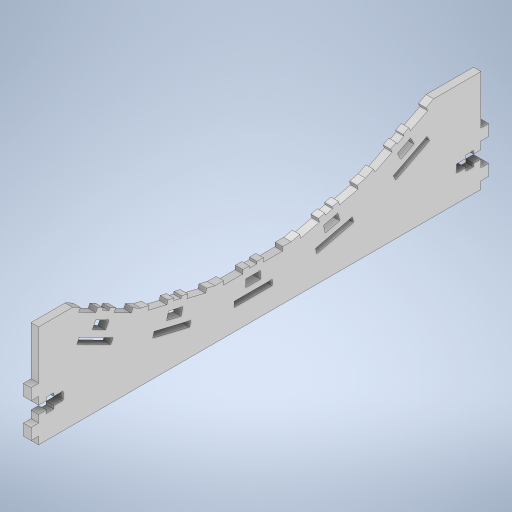
# Autodesk Inventor part: switchplate-support-03
Saved by Autodesk Inventor 2024.1 (Build 281209000, 209)
## iProperties
Created: 2019-06-27
Material: Acier, galvanisé
Document SubType Name: Modeling
Designer: Thibault
Density: 7.85 g/cm^3
Appearance: Aluminium - Poli
Mass: 11.7255 g
Surface Area: 33.7109 cm^2
Volume: 1.4937 cm^3
Part Number: switchplate-support-03
sa_0: 0.400 nd
height_shift: 0,000 mm
base_height: 27,000 mm
switchplate_depth: 121,000 mm
short_switchplate_depth: 96,505 mm
Author: Thibault
Autodesk Inventor part; units mm, degrees
ref_plane "YZ Plane" through (0, 0, 0) normal (1, 0, 0) x (0, 1, 0)
ref_plane "XZ Plane" through (0, 0, 0) normal (0, 1, 0) x (-1, 0, 0)
ref_plane "XY Plane" through (0, 0, 0) normal (0, 0, 1) x (1, 0, 0)
sketch "Anchor (nut side)" plane through (0, 0, 0) normal (0, 0, 1) x (1, 0, 0)
  line L0 (11.1, 0) -> (9.1, 0)
  line L1 (9.1, 0) -> (9.1, -2)
  line L2 (9.1, -2) -> (9.9, -2)
  line L3 (9.9, -2) -> (9.9, -4)
  line L4 (6.2, -4) -> (6.2, -2)
  line L5 (6.2, -2) -> (7, -2)
  line L6 (7, -2) -> (7, 0)
  line L7 (7, 0) -> (5, 0)
  line L8 (2, 0) -> (2, 2)
  line L9 (2, 0) -> (3, 0) construction
  line L10 (2, 2) -> (5, 2)
  line L11 (5, 2) -> (5, 0)
  line L12 (11.1, 0) -> (11.1, 2)
  line L13 (11.1, 2) -> (14.1, 2)
  line L14 (14.1, 2) -> (14.1, 0)
  line L15 (0, 0) -> (2, 0)
  line L16 (14.1, 0) -> (16.1, 0)
  line L17 (6.2, -4) -> (7, -4)
  line L18 (9.9, -4) -> (9.1, -4)
  line L19 (7, -4) -> (7, -6.25)
  line L20 (9.1, -4) -> (9.1, -6.25)
  line L21 (7.25, -6.5) -> (8.05, -6.5)
  arc A0 (7, -6.25) -> (7.25, -6.5) centre (7.25, -6.25) ccw
  arc A1 (8.85, -6.5) -> (9.1, -6.25) centre (8.85, -6.25) ccw
  line L22 (8.05, -6.5) -> (8.85, -6.5)
  line L23 (8.05, -3.8983) -> (8.05, -9.959) construction
  point P0 (9.1321, -0.6227)
  point P1 (7, -6.5)
  point P2 (9.1, -6.5)
  dimension "d3" = 2
  dimension "d7" = 6.1
  dimension "d10" = 2
  dimension "d11" = 2
  dimension "d12" = 0.8
  dimension "d13" = 2
  dimension "d14" = 0.8
  dimension "d15" = 2.1
  dimension "d18" = 2
  dimension "d19" = 0.8
  dimension "d20" = 0.8
  dimension "d21" = 2.5
  dimension "d22" = 2.5
  dimension "d23" = 2.1
  dimension "d38" = 2
  dimension "d39" = 0.25
  dimension "d120" = 3
  measures "d3" distance of point (0, 0) L8.start
  measures "d7" distance of L7.end L0.start
  measures "d10" distance of L0.start L0.end
  measures "d11" distance of L0.end L1.end
  measures "d12" distance of L1.end L2.end
  measures "d13" distance of L2.end L3.end
  measures "d14" distance of L4.end L5.end
  measures "d15" distance of L6.end L0.end
  measures "d18" distance of L14.end point (16.1, 0)
  measures "d19" distance of L4.start L17.end
  measures "d20" distance of L3.end L18.end
  measures "d21" distance of L17.end point (7, -6.5)
  measures "d22" distance of L18.end point (9.1, -6.5)
  measures "d23" distance of L17.end L18.end
  measures "d38" distance of the line from the sketch origin of L10
  measures "d39" radius of A0
  measures "d120" distance of L8.end L10.end
sketch "Anchor (screw side)" plane through (0, 0, 0) normal (0, 0, 1) x (1, 0, 0)
  circle A0 centre (93.8994, 50.2542) radius 1.05
  line L0 (90.8494, 51.2542) -> (87.8494, 51.2542)
  line L1 (87.8494, 51.2542) -> (87.8494, 49.2542)
  line L2 (87.8494, 49.2542) -> (90.8494, 49.2542)
  line L3 (90.8494, 49.2542) -> (90.8494, 51.2542)
  line L4 (99.9494, 51.2542) -> (96.9494, 51.2542)
  line L5 (96.9494, 51.2542) -> (96.9494, 49.2542)
  line L6 (96.9494, 49.2542) -> (99.9494, 49.2542)
  line L7 (99.9494, 49.2542) -> (99.9494, 51.2542)
  line L8 (90.8494, 51.2542) -> (96.9494, 49.2542) construction
  line L9 (96.9494, 51.2542) -> (90.8494, 49.2542) construction
  line L10 (85.8494, 53.2542) -> (101.9494, 53.2542) construction
  line L11 (101.9494, 53.2542) -> (101.9494, 47.2542) construction
  line L12 (101.9494, 47.2542) -> (85.8494, 47.2542) construction
  line L13 (85.8494, 47.2542) -> (85.8494, 53.2542) construction
  point P0 (103.5798, 50.1132)
  dimension "d27_1" = 2.1
  dimension "d28_1" = 3
  dimension "d29" = 2
  dimension "slot_distance" = 6.1
  dimension "d34" = 2
  dimension "d35" = 2
  dimension "d36" = 2
  dimension "d37" = 2
  measures "d27_1" diameter of A0
  measures "d28_1" distance of L2.end L1.end
  measures "d29" distance of L1.end L0.end
  measures "slot_distance" distance between parallel lines of L5 L3
  measures "d34" distance between parallel lines of L0 L10
  measures "d35" distance between parallel lines of L12 L2
  measures "d36" distance between parallel lines of L11 L7
  measures "d37" distance between parallel lines of L13 L1
sketch "Switch support" plane through (0, 0, 0) normal (0, 0, 1) x (1, 0, 0)
  line L0 (15.2854, 16.4472) -> (15.9854, 16.4472)
  line L1 (15.9854, 16.4472) -> (15.9854, 15.4472)
  line L2 (31.5854, 15.4472) -> (31.5854, 16.4472)
  line L3 (31.5854, 16.4472) -> (32.2854, 16.4472)
  line L4 (15.9854, 15.4472) -> (21.0554, 15.4472)
  line L5 (21.0554, 15.4472) -> (21.0554, 16.4472)
  line L6 (21.0554, 16.4472) -> (22.7854, 16.4472)
  line L7 (22.7854, 16.4472) -> (22.7854, 15.8972)
  line L8 (22.7854, 15.8972) -> (24.7854, 15.8972)
  line L9 (24.7854, 15.8972) -> (24.7854, 16.4472)
  line L10 (24.7854, 16.4472) -> (26.5154, 16.4472)
  line L11 (26.5154, 15.4472) -> (26.5154, 16.4472)
  line L12 (26.5154, 15.4472) -> (31.5854, 15.4472)
  line L13 (21.8354, 13.9472) -> (25.7354, 13.9472)
  line L14 (25.7354, 13.9472) -> (25.7354, 11.9472)
  line L15 (25.7354, 11.9472) -> (21.8354, 11.9472)
  line L16 (21.8354, 11.9472) -> (21.8354, 13.9472)
  line L17 (23.7854, 15.8972) -> (23.7854, 13.9472) construction
  line L18 (18.7854, 10.3472) -> (28.7854, 10.3472)
  line L19 (28.7854, 10.3472) -> (28.7854, 8.9472)
  line L20 (28.7854, 8.9472) -> (18.7854, 8.9472)
  line L21 (18.7854, 8.9472) -> (18.7854, 10.3472)
  line L22 (23.7854, 11.9472) -> (23.7854, 10.3472) construction
  point P0 (20.0288, 26.7181)
  point P1 (18.5204, 15.4472)
  dimension "d43" = 1
  dimension "d48" = 17
  dimension "d124" = 0.7
  dimension "d125" = 0.7
  dimension "d126" = 1
  dimension "d127" = 5.07
  dimension "d128" = 1
  dimension "d129" = 1.73
  dimension "d131" = 0.55
  dimension "d132" = 2
  dimension "d133" = 0.55
  dimension "d135" = 1.73
  dimension "d136" = 5.07
  dimension "d137" = 1
  dimension "d138" = 3.9
  dimension "d139" = 2
  dimension "d140" = 1.5
  dimension "d141" = 1.4
  dimension "d142" = 10
  dimension "d143" = 5.1
  measures "d43" distance of L1.start L1.end
  measures "d48" distance of point (32.285, 16.447) point (15.285, 16.447)
  measures "d124" distance of L2.end point (32.285, 16.447)
  measures "d125" distance of point (15.285, 16.447) L1.start
  measures "d126" distance of L2.start L2.end
  measures "d127" distance of L1.end L4.end
  measures "d128" distance of L4.end L5.end
  measures "d129" distance of L5.end L6.end
  measures "d131" distance of L6.end L7.end
  measures "d132" distance of L7.end L8.end
  measures "d133" distance of L8.end L9.end
  measures "d135" distance of L9.end L10.end
  measures "d136" distance of L11.start L2.start
  measures "d137" distance of L11.start L10.end
  measures "d138" distance of L14.end L15.end
  measures "d139" distance of L13.end L14.end
  measures "d140" distance between parallel lines of L13 L4
  measures "d141" distance of L20.end L18.start
  measures "d142" distance of L18.start L18.end
  measures "d143" distance from line of L18 point (18.52, 15.447)
sketch "Sketch1" plane through (0, 0, 0) normal (1, 0, 0) x (0, 1, 0)
  line L0 (0, -121) -> (27, -121)
  line L1 (27, 0) -> (0, 0)
  line L2 (27, -121) -> (27, -106.4804)
  line L3 (26.47, -12.0403) -> (27, -11)
  line L4 (28.2121, -16.9724) -> (22.1003, -16.9724)
  line L5 (26.2736, -12.4256) -> (27, -11)
  line L6 (18.5558, -27.5727) -> (17.8294, -28.9983)
  line L7 (21.9473, -35.6102) -> (15.8356, -35.6102)
  line L8 (17.4559, -30.5541) -> (17.8294, -28.9983)
  line L9 (13.4873, -47.0844) -> (13.1138, -48.6402)
  line L10 (19.8511, -55.1756) -> (13.7394, -55.1756)
  line L11 (13.1138, -50.2402) -> (13.1138, -48.6402)
  line L12 (13.1138, -67.2402) -> (13.1138, -68.8402)
  line L13 (22.0358, -74.7409) -> (15.9241, -74.7409)
  line L14 (13.4873, -70.396) -> (13.1138, -68.8402)
  line L15 (17.4559, -86.9263) -> (17.8294, -88.4821)
  line L16 (28.3566, -93.3787) -> (22.2449, -93.3787)
  line L17 (18.5558, -89.9077) -> (17.8294, -88.4821)
  line L18 (26.2736, -105.0548) -> (27, -106.4804)
  line L19 (27, 0) -> (27, -11)
  line L20 (0, 0) -> (0, -121)
  line L21 (17.4559, -30.5541) -> (17.2925, -31.2348)
  line L22 (17.2925, -31.2348) -> (16.3201, -31.0013)
  line L23 (12.6783, -46.1703) -> (13.6507, -46.4038)
  line L24 (13.6507, -46.4038) -> (13.4873, -47.0844)
  line L25 (16.3201, -31.0013) -> (15.1365, -35.9313)
  line L26 (15.1365, -35.9313) -> (16.1089, -36.1647)
  line L27 (16.1089, -36.1647) -> (15.705, -37.8469)
  line L28 (15.705, -37.8469) -> (15.1702, -37.7185)
  line L29 (15.1702, -37.7185) -> (14.7033, -39.6632)
  line L30 (14.7033, -39.6632) -> (15.2381, -39.7916)
  line L31 (15.2381, -39.7916) -> (14.8343, -41.4738)
  line L32 (13.8619, -41.2404) -> (14.8343, -41.4738)
  line L33 (13.8619, -41.2404) -> (12.6783, -46.1703)
  line L34 (13.4959, -36.3395) -> (12.5855, -40.1318)
  line L35 (12.5855, -40.1318) -> (10.6407, -39.6649)
  line L36 (10.6407, -39.6649) -> (11.5511, -35.8726)
  line L37 (11.5511, -35.8726) -> (13.4959, -36.3395)
  line L38 (14.9368, -38.6909) -> (13.0407, -38.2357) construction
  line L39 (10.7074, -32.5334) -> (8.3729, -42.2571)
  line L40 (8.3729, -42.2571) -> (7.0116, -41.9303)
  line L41 (7.0116, -41.9303) -> (9.346, -32.2066)
  line L42 (9.346, -32.2066) -> (10.7074, -32.5334)
  line L43 (11.0959, -37.7688) -> (9.5401, -37.3953) construction
  line L44 (26.2736, -12.4256) -> (25.9558, -13.0493)
  line L45 (25.9558, -13.0493) -> (25.0648, -12.5953)
  line L46 (17.9826, -26.495) -> (18.8736, -26.949)
  line L47 (18.8736, -26.949) -> (18.5558, -27.5727)
  line L48 (25.0648, -12.5953) -> (22.7631, -17.1127)
  line L49 (22.7631, -17.1127) -> (23.6541, -17.5667)
  line L50 (23.6541, -17.5667) -> (22.8687, -19.1082)
  line L51 (22.8687, -19.1082) -> (22.3786, -18.8585)
  line L52 (22.3786, -18.8585) -> (21.4707, -20.6405)
  line L53 (21.4707, -20.6405) -> (21.9607, -20.8902)
  line L54 (21.9607, -20.8902) -> (21.1753, -22.4316)
  line L55 (20.2843, -21.9776) -> (21.1753, -22.4316)
  line L56 (20.2843, -21.9776) -> (17.9826, -26.495)
  line L57 (21.0725, -17.1267) -> (19.3019, -20.6017)
  line L58 (19.3019, -20.6017) -> (17.5199, -19.6937)
  line L59 (17.5199, -19.6937) -> (19.2904, -16.2187)
  line L60 (19.2904, -16.2187) -> (21.0725, -17.1267)
  line L61 (21.9246, -19.7495) -> (20.1872, -18.8642) construction
  line L62 (19.2495, -12.7748) -> (14.7096, -21.6849)
  line L63 (14.7096, -21.6849) -> (13.4622, -21.0493)
  line L64 (13.4622, -21.0493) -> (18.0021, -12.1392)
  line L65 (18.0021, -12.1392) -> (19.2495, -12.7748)
  line L66 (18.4052, -17.9562) -> (16.9796, -17.2298) construction
  line L67 (13.1138, -50.2402) -> (13.1138, -50.9402)
  line L68 (13.1138, -50.9402) -> (12.1138, -50.9402)
  line L69 (12.1138, -66.5402) -> (13.1138, -66.5402)
  line L70 (13.1138, -66.5402) -> (13.1138, -67.2402)
  line L71 (12.1138, -50.9402) -> (12.1138, -56.0102)
  line L72 (12.1138, -56.0102) -> (13.1138, -56.0102)
  line L73 (13.1138, -56.0102) -> (13.1138, -57.7402)
  line L74 (13.1138, -57.7402) -> (12.5638, -57.7402)
  line L75 (12.5638, -57.7402) -> (12.5638, -59.7402)
  line L76 (12.5638, -59.7402) -> (13.1138, -59.7402)
  line L77 (13.1138, -59.7402) -> (13.1138, -61.4702)
  line L78 (12.1138, -61.4702) -> (13.1138, -61.4702)
  line L79 (12.1138, -61.4702) -> (12.1138, -66.5402)
  line L80 (10.6138, -56.7902) -> (10.6138, -60.6902)
  line L81 (10.6138, -60.6902) -> (8.6138, -60.6902)
  line L82 (8.6138, -60.6902) -> (8.6138, -56.7902)
  line L83 (8.6138, -56.7902) -> (10.6138, -56.7902)
  line L84 (12.5638, -58.7402) -> (10.6138, -58.7402) construction
  line L85 (7.0138, -53.7402) -> (7.0138, -63.7402)
  line L86 (7.0138, -63.7402) -> (5.6138, -63.7402)
  line L87 (5.6138, -63.7402) -> (5.6138, -53.7402)
  line L88 (5.6138, -53.7402) -> (7.0138, -53.7402)
  line L89 (8.6138, -58.7402) -> (7.0138, -58.7402) construction
  line L90 (13.4873, -70.396) -> (13.6507, -71.0767)
  line L91 (13.6507, -71.0767) -> (12.6783, -71.3101)
  line L92 (16.3201, -86.4791) -> (17.2925, -86.2456)
  line L93 (17.2925, -86.2456) -> (17.4559, -86.9263)
  line L94 (12.6783, -71.3101) -> (13.8619, -76.24)
  line L95 (13.8619, -76.24) -> (14.8343, -76.0066)
  line L96 (14.8343, -76.0066) -> (15.2381, -77.6888)
  line L97 (15.2381, -77.6888) -> (14.7033, -77.8172)
  line L98 (14.7033, -77.8172) -> (15.1702, -79.7619)
  line L99 (15.1702, -79.7619) -> (15.705, -79.6335)
  line L100 (15.705, -79.6335) -> (16.1089, -81.3157)
  line L101 (15.1365, -81.5492) -> (16.1089, -81.3157)
  line L102 (15.1365, -81.5492) -> (16.3201, -86.4791)
  line L103 (12.5855, -77.3486) -> (13.4959, -81.1409)
  line L104 (13.4959, -81.1409) -> (11.5511, -81.6078)
  line L105 (11.5511, -81.6078) -> (10.6407, -77.8155)
  line L106 (10.6407, -77.8155) -> (12.5855, -77.3486)
  line L107 (14.9368, -78.7895) -> (13.0407, -79.2448) construction
  line L108 (8.3729, -75.2233) -> (10.7074, -84.947)
  line L109 (10.7074, -84.947) -> (9.346, -85.2738)
  line L110 (9.346, -85.2738) -> (7.0116, -75.5501)
  line L111 (7.0116, -75.5501) -> (8.3729, -75.2233)
  line L112 (11.0959, -79.7116) -> (9.5401, -80.0852) construction
  line L113 (18.5558, -89.9077) -> (18.8736, -90.5314)
  line L114 (18.8736, -90.5314) -> (17.9826, -90.9854)
  line L115 (25.0648, -104.8851) -> (25.9558, -104.4311)
  line L116 (25.9558, -104.4311) -> (26.2736, -105.0548)
  line L117 (17.9826, -90.9854) -> (20.2843, -95.5028)
  line L118 (20.2843, -95.5028) -> (21.1753, -95.0488)
  line L119 (21.1753, -95.0488) -> (21.9607, -96.5902)
  line L120 (21.9607, -96.5902) -> (21.4707, -96.8399)
  line L121 (21.4707, -96.8399) -> (22.3786, -98.6219)
  line L122 (22.3786, -98.6219) -> (22.8687, -98.3722)
  line L123 (22.8687, -98.3722) -> (23.6541, -99.9137)
  line L124 (22.7631, -100.3677) -> (23.6541, -99.9137)
  line L125 (22.7631, -100.3677) -> (25.0648, -104.8851)
  line L126 (19.3019, -96.8788) -> (21.0725, -100.3537)
  line L127 (21.0725, -100.3537) -> (19.2904, -101.2617)
  line L128 (19.2904, -101.2617) -> (17.5199, -97.7867)
  line L129 (17.5199, -97.7867) -> (19.3019, -96.8788)
  line L130 (21.9246, -97.7309) -> (20.1872, -98.6162) construction
  line L131 (14.7096, -95.7956) -> (19.2495, -104.7056)
  line L132 (19.2495, -104.7056) -> (18.0021, -105.3412)
  line L133 (18.0021, -105.3412) -> (13.4622, -96.4311)
  line L134 (13.4622, -96.4311) -> (14.7096, -95.7956)
  line L135 (18.4052, -99.5242) -> (16.9796, -100.2506) construction
  point P0 (18.5558, -89.9077)
  point P1 (17.4559, -86.9263)
  point P2 (13.1138, -50.2402)
  point P3 (13.4873, -47.0844)
  point P4 (17.4559, -30.5541)
  point P5 (18.5558, -27.5727)
  point P6 (26.2736, -12.4256)
  point P7 (0, -52.3792)
  point P8 (0, -17.4222)
  dimension "height" = 27
  dimension "d193" = 27
  dimension "k1_a" = 1.6
  dimension "k1_b" = 1.6
  dimension "k2_a" = 1.6
  dimension "k2_b" = 1.6
  dimension "k3_a" = 1.6
  dimension "k3_b" = 1.6
  dimension "k4_a" = 1.6
  dimension "k4_b" = 1.6
  dimension "k5_a" = 1.6
  dimension "k5_b" = 1.6
  dimension "d257" = 11
  dimension "d272" = 63
  dimension "d273" = 103.5
  dimension "d274" = 90
  dimension "d275" = 76.5
  dimension "d276" = 63
  constraints: 42 end point, 7 horizontal, 4 vertical, 1 collinear, 1 vertical alignment, 19 other
  measures "height" distance of L1.start L1.end
  measures "d193" distance of L0.end L0.start
  measures "k1_a" distance of L3.end L5.start
  measures "k1_b" distance of L6.end L6.start
  measures "k2_a" distance of L8.start L6.end
  measures "k2_b" distance of L9.end L9.start
  measures "k3_a" distance of L11.start L9.end
  measures "k3_b" distance of L12.end L12.start
  measures "k4_a" distance of L14.start L12.end
  measures "k4_b" distance of L15.end L15.start
  measures "k5_a" distance of L17.start L15.end
  measures "k5_b" distance of L2.end L18.start
  measures "d257" distance of L1.start L3.end
  measures "d274" angle to the sketch y axis of L10
extrude "Base" add sketch "Sketch1" along normal blind 2
sketch "Sketch2" plane through (0, 0, 0) normal (-1, 0, 0) x (0, 0, 1)
  line L0 (-190.1228, 20.337) -> (-190.1228, -18.1383)
  line L1 (129.0949, 104.0572) -> (129.0949, -18.1383)
  line L2 (129.0949, -18.1383) -> (-190.1228, -18.1383)
  line L3 (-121, 0) -> (-121, 0) construction
  line L4 (-119, 16.1) -> (-119, 104.9044)
  line L5 (-119, 104.9044) -> (-190.1228, 104.9044)
  line L6 (-190.1228, 104.9044) -> (-190.1228, 20.337)
  line L7 (-2, 16.1) -> (-2, 104.0572)
  line L8 (-2, 104.0572) -> (129.0949, 104.0572)
  line L9 (0, 27) -> (0, 0) projected
  line L10 (-121, 0) -> (-121, 27) projected
  line L11 (0, 0) -> (-121, 0) projected
  line L12 (-2, 0) -> (-119, 0)
  line L13 (-119, 11.1) -> (-119, 9.1)
  line L14 (-119, 9.1) -> (-117, 9.1)
  line L15 (-117, 9.1) -> (-117, 9.9)
  line L16 (-117, 9.9) -> (-115, 9.9)
  line L17 (-115, 6.2) -> (-117, 6.2)
  line L18 (-117, 6.2) -> (-117, 7)
  line L19 (-117, 7) -> (-119, 7)
  line L20 (-119, 7) -> (-119, 5)
  line L21 (-119, 2) -> (-121, 2)
  line L22 (-119, 2) -> (-119, 3) construction
  line L23 (-121, 2) -> (-121, 5)
  line L24 (-121, 5) -> (-119, 5)
  line L25 (-119, 11.1) -> (-121, 11.1)
  line L26 (-121, 11.1) -> (-121, 14.1)
  line L27 (-121, 14.1) -> (-119, 14.1)
  line L28 (-119, 0) -> (-119, 2)
  line L29 (-119, 14.1) -> (-119, 16.1)
  line L30 (-115, 6.2) -> (-115, 7)
  line L31 (-115, 9.9) -> (-115, 9.1)
  line L32 (-115, 7) -> (-112.75, 7)
  line L33 (-115, 9.1) -> (-112.75, 9.1)
  line L34 (-112.5, 7.25) -> (-112.5, 8.05)
  arc A0 (-112.75, 7) -> (-112.5, 7.25) centre (-112.75, 7.25) ccw
  arc A1 (-112.5, 8.85) -> (-112.75, 9.1) centre (-112.75, 8.85) ccw
  line L35 (-112.5, 8.05) -> (-112.5, 8.85)
  line L36 (-115.1017, 8.05) -> (-109.041, 8.05) construction
  line L37 (-2, 5) -> (-2, 7)
  line L38 (-2, 7) -> (-4, 7)
  line L39 (-4, 7) -> (-4, 6.2)
  line L40 (-4, 6.2) -> (-6, 6.2)
  line L41 (-6, 9.9) -> (-4, 9.9)
  line L42 (-4, 9.9) -> (-4, 9.1)
  line L43 (-4, 9.1) -> (-2, 9.1)
  line L44 (-2, 9.1) -> (-2, 11.1)
  line L45 (-2, 14.1) -> (0, 14.1)
  line L46 (-2, 14.1) -> (-2, 13.1) construction
  line L47 (0, 14.1) -> (0, 11.1)
  line L48 (0, 11.1) -> (-2, 11.1)
  line L49 (-2, 5) -> (0, 5)
  line L50 (0, 5) -> (0, 2)
  line L51 (0, 2) -> (-2, 2)
  line L52 (-2, 16.1) -> (-2, 14.1)
  line L53 (-2, 2) -> (-2, 0)
  line L54 (-6, 9.9) -> (-6, 9.1)
  line L55 (-6, 6.2) -> (-6, 7)
  line L56 (-6, 9.1) -> (-8.25, 9.1)
  line L57 (-6, 7) -> (-8.25, 7)
  line L58 (-8.5, 8.85) -> (-8.5, 8.05)
  arc A2 (-8.25, 9.1) -> (-8.5, 8.85) centre (-8.25, 8.85) ccw
  arc A3 (-8.5, 7.25) -> (-8.25, 7) centre (-8.25, 7.25) ccw
  line L59 (-8.5, 8.05) -> (-8.5, 7.25)
  line L60 (-5.8983, 8.05) -> (-11.959, 8.05) construction
  point P0 (-119, 16.1)
  point P1 (-2, 16.1)
  point P2 (-2, 0)
  constraints: 20 end point, 4 vertical, 3 horizontal, 2 parallel, 1 perpendicular, 4 other
extrude "Standard anchors" cut sketch "Sketch2" against normal through all
sketch "Esquisse7" plane through (0, 0, 0) normal (-1, 0, 0) x (0, 0, 1)
  line L0 (-104.5, 8.35) -> (-102.5, 8.35) construction
  line L1 (-106.5, 9.15) -> (-104.5, 9.15) construction
  line L2 (-104.5, 5.85) -> (-106.5, 5.85) construction
  line L3 (-102.5, 6.65) -> (-104.5, 6.65) construction
  line L4 (-109, 9.15) -> (-100.5, 9.15)
  line L5 (-109, 5.85) -> (-100.5, 5.85)
  line L6 (-109, 10) -> (-109, 8.35) construction
  line L7 (-109, 9.15) -> (-109, 5.85)
  arc A0 (-102.5, 6.65) -> (-102.5, 8.35) centre (-102.5, 7.5) ccw projected
  line L8 (-100.5, 5.85) -> (-100.5, 9.15)
  point P0 (1.5, 20)
  point P1 (108.5, 20)
  point P2 (108.5, 0)
  point P3 (1.5, 0)
  point P4 (-2, 10)
  point P5 (-2, 5)
  point P6 (7.6691, 10.85)
  point P7 (8.8147, 9.7576)
  point P8 (-111, 0)
  point P9 (-102.77, 8.35)
  point P10 (-100.7609, 7.9198)
  dimension "d203" = 2
  constraints: 8 end point, 2 collinear, 1 perpendicular, 1 vertical, 2 other
  measures "d203" distance from line of L8 A0.centre
extrude "No back screw hole" [suppressed]
sketch "Esquisse13" plane through (2, 0, 0) normal (1, 0, 0) x (0, 0, -1)
  line L0 (19.7689, 15.7099) -> (20.8292, 18.6229)
  line L1 (20.8292, 18.6229) -> (22.8025, 17.9047)
  line L2 (22.8025, 17.9047) -> (21.7423, 14.9916)
  line L3 (21.7423, 14.9916) -> (19.7689, 15.7099)
  line L4 (22.8025, 17.9047) -> (21.7423, 14.9916) projected
  line L5 (19.7689, 15.7099) -> (20.8292, 18.6229) projected
  line L6 (20.8292, 18.6229) -> (22.8025, 17.9047) projected
  line L7 (21.7423, 14.9916) -> (19.7689, 15.7099) projected
  point P0 (0, 0)
  constraints: 8 end point, 4 collinear
extrude "Hole fixup" [suppressed]
sketch "Esquisse8" plane through (0, 0, 0) normal (-1, 0, 0) x (0, 0, 1)
  line L0 (0, 0) -> (-100.5509, 0) projected
  line L1 (0, 0) -> (-20.4545, 0)
  line L2 (0, 66.4589) -> (0, 0)
  line L3 (0, 27) -> (0, 0) projected
  line L4 (-26.495, 66.4589) -> (0, 66.4589)
  line L5 (-26.495, 66.4589) -> (-26.495, 16.1)
  line L6 (-121, 2) -> (-121, 27) projected
  line L7 (-26.495, 5) -> (-26.495, 7)
  line L8 (-26.495, 7) -> (-28.495, 7)
  line L9 (-28.495, 7) -> (-28.495, 6.2)
  line L10 (-28.495, 6.2) -> (-30.495, 6.2)
  line L11 (-30.495, 9.9) -> (-28.495, 9.9)
  line L12 (-28.495, 9.9) -> (-28.495, 9.1)
  line L13 (-28.495, 9.1) -> (-26.495, 9.1)
  line L14 (-26.495, 9.1) -> (-26.495, 11.1)
  line L15 (-26.495, 14.1) -> (-24.495, 14.1)
  line L16 (-26.495, 14.1) -> (-26.495, 13.1) construction
  line L17 (-24.495, 14.1) -> (-24.495, 11.1)
  line L18 (-24.495, 11.1) -> (-26.495, 11.1)
  line L19 (-26.495, 5) -> (-24.495, 5)
  line L20 (-24.495, 5) -> (-24.495, 2)
  line L21 (-24.495, 2) -> (-26.495, 2)
  line L22 (-26.495, 16.1) -> (-26.495, 14.1)
  line L23 (-26.495, 2) -> (-26.495, 0)
  line L24 (-30.495, 9.9) -> (-30.495, 9.1)
  line L25 (-30.495, 6.2) -> (-30.495, 7)
  line L26 (-30.495, 9.1) -> (-32.745, 9.1)
  line L27 (-30.495, 7) -> (-32.745, 7)
  line L28 (-32.995, 8.85) -> (-32.995, 8.05)
  arc A0 (-32.745, 9.1) -> (-32.995, 8.85) centre (-32.745, 8.85) ccw
  arc A1 (-32.995, 7.25) -> (-32.745, 7) centre (-32.745, 7.25) ccw
  line L29 (-32.995, 8.05) -> (-32.995, 7.25)
  line L30 (-30.3933, 8.05) -> (-36.454, 8.05) construction
  point P0 (110, 0)
  point P1 (-109, 0)
  point P2 (-121, 0)
  point P3 (0, 12.75)
  point P4 (0, 10.25)
  point P5 (0, 12)
  point P6 (-26.495, 0)
  point P7 (-121, 5)
  point P8 (-26.495, 17.9826)
  dimension "d232" = 20.4545
  constraints: 8 end point, 3 vertical, 2 collinear, 2 horizontal, 1 parallel, 1 point on line, 1 other
  measures "d232" distance of L0.start L1.end
extrude "Short plate" [suppressed]
derived "shared_parameters.ipt"
equation "\"depth_shift\" = 5"
equation "\"angle\" = 13.5deg"
equation "\"a_default\" = 1.6"
equation "\"b_default\" = 1.6"
